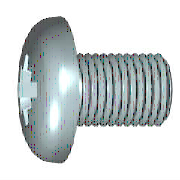
# Autodesk Inventor part: BS 4183 - M8 x 35
Saved by Autodesk Inventor 2022 (Build 260153000, 153)
## iProperties
Created: 2021-02-02
Part Number: BS 4183 - M8 x 35
Material: Сталь, мягкая
Description: Винты и гайки крепежные мелкие. Метрическая серия
Document SubType Name: Modeling
Standard: BS 4183
Designer: Petrov Ivan
Standards Organization: BSI
Language: ru-RU
Size Designation: M8 x 35
Categories: <MemberInstance><Categories><Category DisplayName="Крепежные изделия" InternalName="e4da775c-781d-43d5-af7c-5136215cf5a6" Mnemonic="FSTN"><Category DisplayName="Болты  Винты" InternalName="536e6df0-f778-49ac-b2f2-25c71d2aa0b2" Mnemonic="SCRW"><CategoryParameter DisplayName="Обозначение номинального диаметра" InternalName="03caf894-eafd-4c09-a035-916ac084b87b" Mnemonic="nomdiadesig"/><CategoryParameter DisplayName="Номинальная длина" InternalName="238ecbaf-3e6c-45dd-aa95-4068c8e0fd02" Mnemonic="nomlen"/><CategoryParameter DisplayName="Обозначение резьбы" InternalName="586d5e89-370a-4089-914f-0110033585c7" Mnemonic="thrdesign"/><CategoryParameter DisplayName="Обозначение серии резьб" InternalName="87c5849c-b3a5-4c3e-9c9b-2feecef9be86" Mnemonic="thrserdsgn"/><CategoryParameter DisplayName="Номинальный диаметр" InternalName="8bbe3f8e-44cf-40a9-a251-3a6edc8168d6" Mnemonic="nomdia"/><CategoryParameter DisplayName="Тип резьбы" InternalName="b4bbb7bc-d6aa-4c9f-a9a9-4152b9f6fe49" Mnemonic="thrtype"/><CategoryParameter DisplayName="Шаг резьбы" InternalName="bb82302e-82d8-4176-8fc1-c5d7bb17d5ad" Mnemonic="pitch1"/><CategoryParameter DisplayName="Витков на единицу" InternalName="bdc6e7d2-ffd0-4d9c-a173-16b95ebb912d" Mnemonic="thrperunit1"/><CategoryParameter DisplayName="Класс резьбы" InternalName="ebc0d23b-2cc6-4d2a-b376-d52aae53bab6" Mnemonic="thrclss"/><Category DisplayName="С полукруглой головкой" InternalName="df3578aa-538f-4805-96a8-2439eb0c3cf7" Mnemonic="RNDSCRW"><CategoryParameter DisplayName="Длина стержня" InternalName="2c6ace26-543b-4217-91c4-9cdf8c3ec6f1" Mnemonic="grplen"/><CategoryParameter DisplayName="Высота головки" InternalName="2d152238-84fe-49ae-94c3-3fee884c292b" Mnemonic="headh"/><CategoryParameter DisplayName="Квалитет" InternalName="85496db6-1567-48ed-b0d4-aa1f03366005" Mnemonic="propclss"/><CategoryParameter DisplayName="Длина резьбы" InternalName="a1e5edc5-4ca7-4847-8786-65b14d35af16" Mnemonic="thrlen"/><CategoryParameter DisplayName="Диаметр стержня" InternalName="c22f1a48-b8d5-43ef-ac5e-546ba91c0bd6" Mnemonic="grpdia"/><CategoryParameter DisplayName="Диаметр головки" InternalName="e71ee7a1-06fd-425c-ba3b-09769885677c" Mnemonic="headdia"/></Category></Category></Category><Category DisplayName="ТипДанных" InternalName="23b78d0f-2648-40c6-8793-ca6db495c9e8" Mnemonic="DATATYPE"><CategoryParameter DisplayName="ОтображаемоеИмя" InternalName="05415f3d-3907-474b-a020-eb9d644f4cf3" Mnemonic="DISPLAYNAME"/><CategoryParameter DisplayName="Стандарт" InternalName="0c0a119c-1e12-4c84-803f-101930972f5e" Mnemonic="STANDARD"/><CategoryParameter DisplayName="Наименование" InternalName="13903e3d-64b1-4950-80da-f627842ea37f" Mnemonic="DESCRIPTION"/><CategoryParameter DisplayName="Обозначение" InternalName="2675968c-4ce5-49e0-a4f5-552d29089031" Mnemonic="DESIGNATION"/><CategoryParameter DisplayName="Строка по умолчанию" InternalName="2af9ec52-faaa-4026-b378-f9fa4afca842" Mnemonic="DEFAULTROW"/><CategoryParameter DisplayName="Имя папки" InternalName="3f06958e-8713-4116-9be7-ed6184ecc97b" Mnemonic="FOLDERNAME"/><CategoryParameter DisplayName="Указатель редакций" InternalName="45a75005-10b1-4dfc-8d6d-dfe629f0b93c" Mnemonic="REVISIONGUID"/><CategoryParameter DisplayName="ИмяФайла" InternalName="8b46a4cc-9585-4fed-90c3-899f57e09a73" Mnemonic="FILENAME"/><CategoryParameter DisplayName="ОргСтанд" InternalName="8f5914e1-4693-403f-8ab5-d37768198c9d" Mnemonic="STDSORG"/><CategoryParameter DisplayName="Версия семейства" InternalName="914462f6-6e19-4b14-ba84-155b9680b1d0" Mnemonic="FAMILYREVISION"/><CategoryParameter DisplayName="Редакция стандарта" InternalName="91d5a463-65c2-4fde-b823-3b7fea5e8e17" Mnemonic="STANDARDREVISION"/><CategoryParameter DisplayName="редакция элемента" InternalName="a65d44b9-392f-4f4f-857b-e4b3d54996fe" Mnemonic="MEMBERREVISION"/><CategoryParameter DisplayName="ФорматКлипа" InternalName="bc51e27b-3422-4e78-93ef-cec197ddf230" Mnemonic="CLIPFORMAT"/><CategoryParameter DisplayName="Изготовитель" InternalName="cd6c7a72-a28a-4e50-99a9-2c7f4e13e5ad" Mnemonic="MANUFACTURER"/><CategoryParameter DisplayName="ВнутреннееИмя" InternalName="cf1d0246-76d9-4b4a-8305-fa0409afb5c1" Mnemonic="INTERNALNAME"/><CategoryParameter DisplayName="Метрическая" InternalName="e2385c5b-1ea4-4823-96a8-8de651266ec3" Mnemonic="ISMETRIC"/><Category DisplayName="Деталь" InternalName="c0e0b642-3bcb-4cc8-9e80-f96d35c4afa4" Mnemonic="PART"><CategoryParameter DisplayName="Номер детали" InternalName="016b6077-bfbe-49bd-92c9-d8d59c39c941" Mnemonic="PARTNUMBER"/><CategoryParameter DisplayName="Инвентарный номер" InternalName="4dba7c1c-e26c-444e-836c-b08b433409a8" Mnemonic="STOCKNUMBER"/><CategoryParameter DisplayName="Ключ материала" InternalName="5c9a8adb-dd2b-4535-b97f-0a94a95fe41f" Mnemonic="MATERIALKEY"/><CategoryParameter DisplayName="Материал" InternalName="818a152a-d3c3-49ca-80ee-df7d91421b8e" Mnemonic="MATERIAL"/></Category></Category><Category DisplayName="СтараяКарта" InternalName="cd87c42b-3e48-431e-b5c0-1cbeb14dfe77" Mnemonic="LEGACYMAP"><CategoryParameter DisplayName="уникальное обозначение элемента DA" InternalName="0918ad47-427f-4fed-ae26-24c81c58f590" Mnemonic="DACOOKIE"/><CategoryParameter DisplayName="Объединить код 11" InternalName="0ee8fb18-e2ed-4f39-96f6-1f4b5f50aa71" Mnemonic="MERGE11"/><CategoryParameter DisplayName="уникальное обозначение элемента CC" InternalName="5193edd4-b2b0-4ab4-9d54-de900eee34e0" Mnemonic="CCCOOKIE"/><CategoryParameter DisplayName="Разделить код" InternalName="72b5c83c-be7f-45c4-ae51-9160ea6deb26" Mnemonic="SPLIT"/><CategoryParameter DisplayName="КодУчастника" InternalName="8e5e0294-fc51-4c8f-b3d7-003dc5ed94f6" Mnemonic="MEMBERID"/><CategoryParameter DisplayName="ИмяКаталога" InternalName="d99d1e27-aa94-4de2-af4c-c348882a6f4f" Mnemonic="CATALOGNAME"/><CategoryParameter DisplayName="НомерСемейства" InternalName="e705e1f4-09cb-413e-91f9-551b4188271e" Mnemonic="FAMILYNUMBER"/></Category></Categories><FamilyTemplate Id="si0152"><FamilyTemplateParameters><FamilyTemplateParameter ObjectType="kUserParameterObject" ValueType="xs:double" Id="1" ObjectReferenceKey="GUL"/><FamilyTemplateParameter ObjectType="kUserParameterObject" ValueType="xs:double" Id="2" ObjectReferenceKey="SPD"/><FamilyTemplateParameter ObjectType="kUserParameterObject" ValueType="xs:double" Id="3" ObjectReferenceKey="NLG"/><FamilyTemplateParameter ObjectType="kUserParameterObject" ValueType="xs:double" Id="4" ObjectReferenceKey="KOD"/><FamilyTemplateParameter ObjectType="kUserParameterObject" ValueType="xs:double" Id="5" ObjectReferenceKey="SBR"/><FamilyTemplateParameter ObjectType="kUserParameterObject" ValueType="xs:double" Id="6" ObjectReferenceKey="KR"/><FamilyTemplateParameter ObjectType="kUserParameterObject" ValueType="xs:double" Id="7" ObjectReferenceKey="PTC"/><FamilyTemplateParameter ObjectType="kUserParameterObject" ValueType="xs:double" Id="8" ObjectReferenceKey="GEL"/><FamilyTemplateParameter ObjectType="kUserParameterObject" ValueType="xs:double" Id="9" ObjectReferenceKey="THREADDIA"/><FamilyTemplateParameter ObjectType="kUserParameterObject" ValueType="xs:double" Id="10" ObjectReferenceKey="TOA"/><FamilyTemplateParameter ObjectType="kUserParameterObject" ValueType="xs:double" Id="11" ObjectReferenceKey="BDM"/><FamilyTemplateParameter ObjectType="kUserParameterObject" ValueType="xs:double" Id="12" ObjectReferenceKey="RR"/><FamilyTemplateParameter ObjectType="kUserParameterObject" ValueType="xs:double" Id="13" ObjectReferenceKey="STI"/><FamilyTemplateParameter ObjectType="kUserParameterObject" ValueType="xs:double" Id="14" ObjectReferenceKey="TPU"/><FamilyTemplateParameter ObjectType="kUserParameterObject" ValueType="xs:double" Id="15" ObjectReferenceKey="KOH"/><FamilyTemplateParameter ObjectType="kUserParameterObject" ValueType="xs:double" Id="16" ObjectReferenceKey="SDM"/><FamilyTemplateParameter ObjectType="kUserParameterObject" ValueType="xs:double" Id="17" ObjectReferenceKey="NND"/><FamilyTemplateParameter ObjectType="kUserParameterObject" ValueType="xs:double" Id="18" ObjectReferenceKey="GD"/><FamilyTemplateParameter ObjectType="kUserParameterObject" ValueType="xs:double" Id="19" ObjectReferenceKey="GAL"/><FamilyTemplateParameter ObjectType="kUserParameterObject" ValueType="xs:double" Id="20" ObjectReferenceKey="KEWI"/><FamilyTemplateParameter ObjectType="kUserParameterObject" ValueType="xs:double" Id="21" ObjectReferenceKey="GD1"/><FamilyTemplateParameter ObjectType="kPropertyObject" ValueType="xs:string" Id="100" ObjectReferenceKey="{32853F0F-3444-11d1-9E93-0060B03C1CA6}" SubObjectId="52"/><FamilyTemplateParameter ObjectType="kPropertyObject" ValueType="xs:string" Id="105" ObjectReferenceKey="{32853F0F-3444-11d1-9E93-0060B03C1CA6}" SubObjectId="5"/><FamilyTemplateParameter ObjectType="kPartComponentDefinitionObject" ValueType="xs:string" Id="110" SubObjectId="Material"/><FamilyTemplateParameter ObjectType="kThreadFeatureObject" ValueType="xs:structure" Id="300" ObjectReferenceKey="1002000010000000aa0f0000000000008000000000000000" SubObjectId="ThreadInfo"><FamilyTemplateParameter ObjectType="" ValueType="xs:string" Id="301" SubObjectId="ThreadDesignation"/><FamilyTemplateParameter ObjectType="" ValueType="xs:string" Id="302" SubObjectId="ThreadType"/><FamilyTemplateParameter ObjectType="" ValueType="xs:string" Id="303" SubObjectId="ThreadClass"/></FamilyTemplateParameter></FamilyTemplateParameters></FamilyTemplate><CategoryParameterMap><ParamToTemplateMap><ParamToTemplate CategoryParameter="//CategoryParameter[@InternalName='05415f3d-3907-474b-a020-eb9d644f4cf3']" ConstantValue="BS 4183 Specification for machine screws and machine screw nuts. Metric series - Metric"/><ParamToTemplate CategoryParameter="//CategoryParameter[@InternalName='cf1d0246-76d9-4b4a-8305-fa0409afb5c1']" ConstantValue="8519f130-5df3-44a2-871f-baca5fb80742"/><ParamToTemplate CategoryParameter="//CategoryParameter[@InternalName='3f06958e-8713-4116-9be7-ed6184ecc97b']" ConstantValue="BS 4183(4)"/><ParamToTemplate CategoryParameter="//CategoryParameter[@InternalName='914462f6-6e19-4b14-ba84-155b9680b1d0']" ConstantValue="10"/><ParamToTemplate CategoryParameter="//CategoryParameter[@InternalName='bc51e27b-3422-4e78-93ef-cec197ddf230']" ConstantValue="CF_INVENTOR.STDPARTS"/><ParamToTemplate CategoryParameter="//CategoryParameter[@InternalName='e2385c5b-1ea4-4823-96a8-8de651266ec3']" ConstantValue="true"/><ParamToTemplate CategoryParameter="//CategoryParameter[@InternalName='13903e3d-64b1-4950-80da-f627842ea37f']" ConstantValue="Specification for machine screws and machine screw nuts. Metric series"/><ParamToTemplate CategoryParameter="//CategoryParameter[@InternalName='8f5914e1-4693-403f-8ab5-d37768198c9d']" ConstantValue="BSI"/><ParamToTemplate CategoryParameter="//CategoryParameter[@InternalName='0c0a119c-1e12-4c84-803f-101930972f5e']" ConstantValue="BS 4183"/><ParamToTemplate CategoryParameter="//CategoryParameter[@InternalName='cd6c7a72-a28a-4e50-99a9-2c7f4e13e5ad']" TemplateParameter="104"/><ParamToTemplate CategoryParameter="//CategoryParameter[@InternalName='91d5a463-65c2-4fde-b823-3b7fea5e8e17']" TemplateParameter="103"/><ParamToTemplate CategoryParameter="//CategoryParameter[@InternalName='45a75005-10b1-4dfc-8d6d-dfe629f0b93c']" ConstantValue="3aa5c503-b9d1-43e2-bda9-c368d3b0c4ec"/><ParamToTemplate CategoryParameter="//CategoryParameter[@InternalName='2af9ec52-faaa-4026-b378-f9fa4afca842']" ConstantValue="10"/><ParamToTemplate CategoryParameter="//CategoryParameter[@InternalName='d99d1e27-aa94-4de2-af4c-c348882a6f4f']" ConstantValue="BSI"/><ParamToTemplate CategoryParameter="//CategoryParameter[@InternalName='e705e1f4-09cb-413e-91f9-551b4188271e']" ConstantValue="14"/><ParamToTemplate CategoryParameter="//CategoryParameter[@InternalName='8b46a4cc-9585-4fed-90c3-899f57e09a73']" ConstantValue="BS 4183 - M8 x 35(1) III"/><ParamToTemplate CategoryParameter="//CategoryParameter[@InternalName='a65d44b9-392f-4f4f-857b-e4b3d54996fe']" ConstantValue="D72F07D6-1684-4968-8698-4BF217A3A903"/><ParamToTemplate CategoryParameter="//CategoryParameter[@InternalName='2c6ace26-543b-4217-91c4-9cdf8c3ec6f1']" ConstantValue="2,5"/><ParamToTemplate CategoryParameter="//CategoryParameter[@InternalName='ebc0d23b-2cc6-4d2a-b376-d52aae53bab6']" ConstantValue="6g"/><ParamToTemplate CategoryParameter="//CategoryParameter[@InternalName='03caf894-eafd-4c09-a035-916ac084b87b']" ConstantValue="M8"/><ParamToTemplate CategoryParameter="//CategoryParameter[@InternalName='b4bbb7bc-d6aa-4c9f-a9a9-4152b9f6fe49']" ConstantValue="ISO Metric profile"/><ParamToTemplate CategoryParameter="//CategoryParameter[@InternalName='8e5e0294-fc51-4c8f-b3d7-003dc5ed94f6']" ConstantValue="1290"/><ParamToTemplate CategoryParameter="//CategoryParameter[@InternalName='c22f1a48-b8d5-43ef-ac5e-546ba91c0bd6']" TemplateParameter="11"/><ParamToTemplate CategoryParameter="//CategoryParameter[@InternalName='2675968c-4ce5-49e0-a4f5-552d29089031']" TemplateParameter="100"/><ParamToTemplate CategoryParameter="//CategoryParameter[@InternalName='a1e5edc5-4ca7-4847-8786-65b14d35af16']" TemplateParameter="8"/><ParamToTemplate CategoryParameter="//CategoryParameter[@InternalName='e71ee7a1-06fd-425c-ba3b-09769885677c']" TemplateParameter="4"/><ParamToTemplate CategoryParameter="//CategoryParameter[@InternalName='2d152238-84fe-49ae-94c3-3fee884c292b']" TemplateParameter="15"/><ParamToTemplate CategoryParameter="//CategoryParameter[@InternalName='818a152a-d3c3-49ca-80ee-df7d91421b8e']" TemplateParameter="110"/><ParamToTemplate CategoryParameter="//CategoryParameter[@InternalName='238ecbaf-3e6c-45dd-aa95-4068c8e0fd02']" TemplateParameter="3"/><ParamToTemplate CategoryParameter="//CategoryParameter[@InternalName='8bbe3f8e-44cf-40a9-a251-3a6edc8168d6']" TemplateParameter="17"/><ParamToTemplate CategoryParameter="//CategoryParameter[@InternalName='016b6077-bfbe-49bd-92c9-d8d59c39c941']" TemplateParameter="105"/><ParamToTemplate CategoryParameter="//CategoryParameter[@InternalName='bb82302e-82d8-4176-8fc1-c5d7bb17d5ad']" TemplateParameter="7"/><ParamToTemplate CategoryParameter="//CategoryParameter[@InternalName='586d5e89-370a-4089-914f-0110033585c7']" TemplateParameter="301"/><ParamToTemplate CategoryParameter="//CategoryParameter[@InternalName='bdc6e7d2-ffd0-4d9c-a173-16b95ebb912d']" TemplateParameter="14"/></ParamToTemplateMap></CategoryParameterMap></MemberInstance>
Density: 7.85 g/cm^3
Appearance: С умеренной полировкой
IsCustomPart: 0
Author: Petrov Ivan
Autodesk Inventor part; units mm, degrees
ref_plane "YZ Plane" through (0, 0, 0) normal (1, 0, 0) x (0, 1, 0)
sketch "Эскиз1" plane through (0, 0, 0) normal (0, 0, 1) x (1, 0, 0)
  line L0 (35, 0) -> (35, 4)
  line L1 (35, 4) -> (2.5, 4)
  line L2 (3.9624, 5.08) -> (3.9624, 5.08)
  arc A0 (-3.1496, 7.7244) -> (-5.6, 0) centre (7.8, 0) ccw
  line L3 (-5.6, 0) -> (-5.6, 7.5101)
  line L4 (-5.0091, 3.9354) -> (-2.6869, 2.7776)
  line L5 (-2.6869, 2.7776) -> (-1.21, 0)
  line L6 (-1.21, 0) -> (35, 0)
  line L7 (-14.4375, 0) -> (43.2396, 0) projected
  line L8 (0, -1.6) -> (0, 9.6) projected
  line L9 (-5.0091, 3.9354) -> (-5.6, 4.23) construction
  line L10 (-3.1496, 7.7244) -> (-5.6, 7.5101)
  line L11 (-3.1496, 7.7244) -> (0, 8)
  line L12 (0, 8) -> (0, 3.6165)
  line L13 (0, 3.6165) -> (1.7332, 3.6165)
  line L14 (1.7332, 3.6165) -> (2.5, 4)
  line L15 (2.5, 4) -> (0, 4) construction
  dimension "d1" = 8
  dimension "d2" = 4.39
  dimension "d16" = 8.46
  dimension "d17" = 62
  dimension "d19" = 26.5
  dimension "d23" = 16
  dimension "d24" = 5
  dimension "d25" = 5.6
  dimension "d26" = 13.4
  dimension "d28" = 7.233
  dimension "d29" = 32.5
  dimension "d30" = 0.7668
  dimension "d31" = 35
  constraints: 28 end point, 5 point on line, 4 collinear, 4 point on circle, 3 parallel, 2 perpendicular, 1 centre point, 1 horizontal, 1 tangent
  measures "d1" diameter of L1 L6
  measures "d2" distance from line of L5.end L3
  measures "d16" diameter of L9.end L6
  measures "d17" angle of L5 L6
  measures "d19" angle of L4 L6
  measures "d23" diameter of L11.end L6
  measures "d24" angle of L11 L6
  measures "d25" distance between parallel lines of L3 L12
  measures "d26" radius of A0
  measures "d28" diameter of L13 L6
  measures "d29" distance of L0.end L1.end
  measures "d30" horizontal distance of L13.end L1.end
  measures "d31" distance between parallel lines of L12 L0
revolve "Базовый элемент" add sketch "Эскиз1" angle 360 about axis through (-1.21, 0, 0) along (1, 0, 0) contours L6 L8 L13 L14 L1 L0 | L6 L5 L4 A0 L11 L8
ref_plane "Work Plane1" through (-5.6, 0, 0) normal (1, 0, 0) x (0, 1, 0)
sketch "Эскиз2" plane through (-5.6, 0, 0) normal (1, 0, 0) x (0, 1, 0)
  circle A0 centre (0, 0) radius 7.7244 projected
  line L0 (-10.8142, 0) -> (10.8142, 0) projected
  line L1 (0, -10.8142) -> (0, 10.8142) projected
  line L2 (0, 4.23) -> (0, 0) construction
  line L3 (0, 0) -> (4.23, 0) construction
  arc A1 (1.692, 0) -> (0, 1.692) centre (0, 0) ccw construction
  line L4 (0, 0) -> (6.7207, 6.7207) construction
  line L5 (1.04, 4.1002) -> (0.6188, 2.0225)
  line L6 (4.1002, 1.04) -> (2.0225, 0.6188)
  arc A2 (0.6188, 2.0225) -> (1.5321, 1.5321) centre (1.1493, 1.9149) ccw
  arc A3 (1.5321, 1.5321) -> (2.0225, 0.6188) centre (1.9149, 1.1493) ccw
  arc A4 (4.23, 0) -> (4.1002, 1.04) centre (0, 0) ccw
  arc A5 (1.04, 4.1002) -> (0, 4.23) centre (0, 0) ccw
  arc A6 (4.1002, 1.04) -> (1.04, 4.1002) centre (0, 0) ccw
  line L7 (1.04, -4.1002) -> (0.6188, -2.0225)
  line L8 (4.1002, -1.04) -> (2.0225, -0.6188)
  arc A7 (1.5321, -1.5321) -> (0.6188, -2.0225) centre (1.1493, -1.9149) ccw
  arc A8 (2.0225, -0.6188) -> (1.5321, -1.5321) centre (1.9149, -1.1493) ccw
  arc A9 (4.1002, -1.04) -> (4.23, 0) centre (0, 0) ccw
  arc A10 (0, -4.23) -> (1.04, -4.1002) centre (0, 0) ccw
  arc A11 (1.04, -4.1002) -> (4.1002, -1.04) centre (0, 0) ccw
  line L9 (-1.04, 4.1002) -> (-0.6188, 2.0225)
  line L10 (-4.1002, 1.04) -> (-2.0225, 0.6188)
  arc A12 (-1.5321, 1.5321) -> (-0.6188, 2.0225) centre (-1.1493, 1.9149) ccw
  arc A13 (-2.0225, 0.6188) -> (-1.5321, 1.5321) centre (-1.9149, 1.1493) ccw
  arc A14 (-4.1002, 1.04) -> (-4.23, 0) centre (0, 0) ccw
  arc A15 (0, 4.23) -> (-1.04, 4.1002) centre (0, 0) ccw
  arc A16 (-1.04, 4.1002) -> (-4.1002, 1.04) centre (0, 0) ccw
  arc A17 (-1.04, -4.1002) -> (0, -4.23) centre (0, 0) ccw
  arc A18 (-4.1002, -1.04) -> (-1.04, -4.1002) centre (0, 0) ccw
  arc A19 (-4.23, 0) -> (-4.1002, -1.04) centre (0, 0) ccw
  line L11 (-4.1002, -1.04) -> (-2.0225, -0.6188)
  line L12 (-1.04, -4.1002) -> (-0.6188, -2.0225)
  arc A20 (-0.6188, -2.0225) -> (-1.5321, -1.5321) centre (-1.1493, -1.9149) ccw
  arc A21 (-1.5321, -1.5321) -> (-2.0225, -0.6188) centre (-1.9149, -1.1493) ccw
  arc A22 (2.115, 0) -> (0, 2.115) centre (0, 0) ccw construction
  dimension "d4" = 45
  dimension "d5" = 3.384
  dimension "d6" = 8.46
  dimension "d7" = 1.04
  dimension "d20" = 4.23
  constraints: 46 point on circle, 25 symmetric about line, 22 centre point, 22 end point, 6 tangent, 4 coincident, 3 collinear, 3 point on line, 1 midpoint, 1 perpendicular, 22 other
  measures "d4" angle of L4 L3
  measures "d5" diameter of A1
  measures "d6" diameter of A6
  measures "d7" distance from line of L5.start L2
  measures "d20" diameter of A22
extrude "Паз" add sketch "Эскиз2" along normal up to next draft 5 contours L6 A3 A2 L5 A6 | A11 L7 A7 A8 L8 | L9 A12 A13 L10 A16 | A18 L11 A21 A20 L12
revolve "Вырез" cut sketch "Эскиз1" angle 360 about axis through (-10, 0, 0) along (1, 0, 0) contours L3 L10 A0
sketch "Эскиз4" plane through (-5.6, 0, 0) normal (1, 0, 0) x (0, 1, 0)
  circle A0 centre (0, 0) radius 7.7244 projected
  line L0 (-10.8142, 0) -> (10.8142, 0) projected
  line L1 (0, -10.8142) -> (0, 10.8142) projected
  line L2 (0, 0) -> (6.4284, 6.4284) construction
  circle A1 centre (0, 0) radius 0.52 construction
  line L3 (0, 0) -> (6.4284, -6.4284) construction
  line L4 (0, 0) -> (-6.4284, 6.4284) construction
  line L5 (0, 0) -> (-6.4284, -6.4284) construction
  line L6 (2.9911, 2.9911) -> (0, 0.52)
  line L7 (-2.9911, 2.9911) -> (-0.52, 0)
  line L8 (-2.9911, -2.9911) -> (0, -0.52)
  line L9 (2.9911, -2.9911) -> (0.52, 0)
  line L10 (2.9911, 2.9911) -> (0.52, 0)
  line L11 (-2.9911, 2.9911) -> (0, 0.52)
  line L12 (-2.9911, -2.9911) -> (-0.52, 0)
  line L13 (2.9911, -2.9911) -> (0, -0.52)
  circle A2 centre (0, 0) radius 4.23 construction
  dimension "d11" = 1.04
  dimension "d14" = 45
  dimension "d35" = 2.9911
  constraints: 24 end point, 10 point on line, 7 point on circle, 3 perpendicular, 3 symmetric about line, 2 centre point, 2 coincident, 3 other
  measures "d11" diameter of A1
  measures "d14" angle of L2 L0
  measures "d35" distance from line of L0 L6.start
extrude "Прорезь крестообразная" cut sketch "Эскиз4" along normal blind 5.6 draft -10 contours L9 L13 L1 L0 | L0 L1 L6 L10 | L1 L0 L7 L11 | L8 L12 L0 L1
fillet "Сопряжение1" radius 3.2 1 edges at (-3.1496, -7.7244, 0)
fillet "Сопряжение2" radius 0.416 5 edges at (-5.0091, 0, 3.9354) (-5.0091, -3.9354, 0) (-5.0091, 0, -3.9354) (-5.0091, 3.9073, 0.4689) (-5.0091, 3.9073, -0.4689)
thread "Резьба" size "M8x1.25" class "6g" standard "ISO Metric profile" length 32.5
chamfer "Фаска1" distance 0.7668 distance2 0.7669 1 edges at (35, -4, 0) measured on face at (35, -3.5, 0)
ref_plane "Work Plane3" through (1.85, 0, 0) normal (0, 1, 0) x (1, 0, 0)
equation "\"d11\" = 0.5 * SBR"
equation "\"d35\" = 0.353553 * SDM"
equation "\"d12\" = KOH"
equation "\"d5\" = 0.4 * SDM"
equation "\"d6\" = SDM"
equation "\"d7\" = 0.5 * SBR"
equation "\"d20\" = 0.5 * SDM"
equation "\"d1\" = GD"
equation "\"d2\" = STI"
equation "\"d16\" = SDM"
equation "\"d23\" = KOD"
equation "\"d24\" = KEWI"
equation "\"d25\" = KOH"
equation "\"d26\" = KR"
equation "\"d28\" = BDM"
equation "\"d29\" = GEL"
equation "\"d30\" = GAL"
equation "\"d31\" = NLG"
equation "\"d32\" = RR"
equation "\"d22\" = 0.2 * SBR"
equation "\"d8\" = GEL"
equation "\"d36\" = -0.5 * SPD + 0.5 * GD"
equation "\"GD\" = NND"
equation "\"NLG\" = 35"
equation "\"GEL\" = 32.5"
equation "\"KOD\" = 2 * NND"
equation "\"KOH\" = 5.6"
equation "\"SDM\" = 8.46"
equation "\"STI\" = 4.39"
equation "\"SBR\" = 2.08"
equation "\"KEWI\" = 5deg"
equation "\"d3\" = -KOH"
equation "\"KR\" = 13.4"
equation "\"BDM\" = 7.233"
equation "\"GAL\" = 0.61345 * PTC"
equation "\"GUL\" = 0.61345 * PTC"
equation "\"RR\" = 3.2"
equation "\"SPD\" = NND - 1.2269 * PTC"
equation "\"PTC\" = 1.25"
equation "\"THREADDIA\" = 8"
equation "\"TOA\" = 30deg"
equation "\"NND\" = 8"
equation "\"GD1\" = THREADDIA - 1.2269 * PTC"
body "Solid1"
